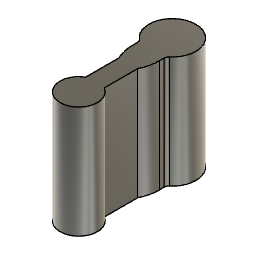
hinge 4 (Autodesk Fusion 360 design; units mm, degrees)
Autodesk Fusion 360 part; units mm, degrees
sketch "Sketch1" plane through (0, 0, 0) normal (0, 0, 1) x (1, 0, 0)
  circle A0 centre (0, 0) radius 3.15
  line L0 (-1.25, -2.8914) -> (-1.25, -10.3914)
  line L1 (1.25, -2.8914) -> (1.25, -10.3914)
  circle A1 centre (0, -12.5564) radius 2.5
  line L2 (-1.25, -5.9082) -> (-1.8, -5.9082)
  line L3 (-1.8, -5.9082) -> (-1.8, -2.5851)
  line L4 (1.25, -5.9082) -> (1.8, -5.9082)
  line L5 (1.8, -5.9082) -> (1.8, -2.5851)
  dimension "d1" = 6.3
  dimension "d2" = 2.5
  dimension "d3" = 1.25
  dimension "d4" = 5
  dimension "d13" = 7.5
  constraint coincident A0.centre origin
  constraint coincident A0 L0.start
  constraint vertical L0
  constraint coincident A0 L1.start
  constraint parallel L0 L1
  constraint coincident L1.end A1
  constraint coincident L0.end A1
  constraint perpendicular L0 L2
  constraint coincident A0 L3.end
  constraint perpendicular L1 L4
  constraint coincident A0 L5.end
  constraint perpendicular L4 L5
  measures "d1" diameter of A0
  measures "d2" distance of L0 L1
  measures "d3" distance of A0.centre L1
  measures "d4" diameter of A1
  measures "d13" distance of L1.start L1.end
extrude "Extrude1" add sketch "Sketch1" along normal blind 15
fillet "Fillet1" radius 0.65 2 edges at (-1.8, -2.5851, 7.5) (1.8, -2.5851, 7.5)
fillet "Fillet2" radius 5.25 1 edges at (1.8, -5.9082, 7.5)
fillet "Fillet3" radius 5.25 1 edges at (-1.8, -5.9082, 7.5)
